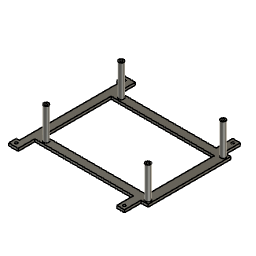
PCB_Rev1_Holder v4 (Autodesk Fusion 360 design; units mm, degrees)
Autodesk Fusion 360 part; units mm, degrees
note: some values were not read from the file. Set by a fixed rule: which face or edge a step refers to.
sketch "Sketch1" plane through (0, 0, 0) normal (0, 0, 1) x (1, 0, 0)
  line L0 (0, 180) -> (180, 180)
  line L1 (180, 180) -> (180, 0)
  line L2 (180, 0) -> (0, 0)
  line L3 (0, 0) -> (0, 180)
  line L4 (10, 170) -> (170, 170)
  line L5 (170, 170) -> (170, 10)
  line L6 (170, 10) -> (10, 10)
  line L7 (10, 10) -> (10, 170)
  constraint horizontal L0
  constraint vertical L1
  constraint horizontal L2
  constraint vertical L3
  constraint horizontal L4
  constraint vertical L5
  constraint horizontal L6
  constraint vertical L7
sketch "Sketch2" plane through (0, 0, 4) normal (0, 0, 1) x (-1, 0, 0)
  line L0 (-170, -10) -> (-10, -10)
  line L1 (-10, -10) -> (-10, -170)
  line L2 (-10, -170) -> (-170, -170)
  line L3 (-170, -170) -> (-170, -10)
  line L4 (0, 0) -> (-180, 0)
  line L5 (-180, 0) -> (-180, -180)
  line L6 (-180, -180) -> (0, -180)
  line L7 (0, -180) -> (0, 0)
  circle A0 centre (-5, -5) radius 2
sketch "Sketch3" plane through (0, 0, 0) normal (0, 0, 1) x (1, 0, 0)
  line L0 (0, 0) -> (172, 0)
  line L1 (172, 0) -> (172, 130)
  line L2 (172, 130) -> (0, 130)
  line L3 (0, 130) -> (0, 0)
  line L4 (12, 12) -> (158, 12)
  line L5 (158, 12) -> (158, 118)
  line L6 (158, 118) -> (12, 118)
  line L7 (12, 118) -> (12, 12)
  dimension "d5" = 172
  dimension "d6" = 130
  constraint horizontal L0
  constraint vertical L1
  constraint horizontal L2
  constraint vertical L3
  constraint coincident L0.start L3.end
  constraint horizontal L4
  constraint vertical L5
  constraint horizontal L6
  constraint vertical L7
  measures "d5" distance of L0.start L0.end
  measures "d6" distance of L0.start L2.end
extrude "Extrude3" add sketch "Sketch3" along normal blind 4
sketch "Sketch4" plane through (0, 0, 4) normal (0, 0, 1) x (-1, 0, 0)
  line L0 (-12, -12) -> (-12, -118)
  line L1 (-12, -118) -> (-158, -118)
  line L2 (-158, -118) -> (-158, -12)
  line L3 (-158, -12) -> (-12, -12)
  line L4 (0, -130) -> (0, 0)
  line L5 (0, 0) -> (-172, 0)
  line L6 (-172, 0) -> (-172, -130)
  line L7 (-172, -130) -> (0, -130)
  circle A0 centre (-6, -6) radius 4
extrude "Extrude4" add sketch "Sketch4" along normal blind 10 contours A0
sketch "Sketch5" plane through (0, 0, 4) normal (0, 0, 1) x (-1, 0, 0)
  circle A0 centre (-6, -6) radius 4
  line L0 (-12, -12) -> (-12, -118)
  line L1 (-12, -118) -> (-158, -118)
  line L2 (-158, -118) -> (-158, -12)
  line L3 (-158, -12) -> (-12, -12)
  line L4 (0, -130) -> (0, 0)
  line L5 (0, 0) -> (-172, 0)
  line L6 (-172, 0) -> (-172, -130)
  line L7 (-172, -130) -> (0, -130)
  circle A1 centre (-6, -124) radius 4
extrude "Extrude5" add sketch "Sketch5" along normal blind 10 contours A1
sketch "Sketch6" plane through (0, 0, 0) normal (0, 0, 1) x (1, 0, 0)
sketch "Sketch7" plane through (0, 0, 4) normal (0, 0, 1) x (-1, 0, 0)
  circle A0 centre (-6, -124) radius 4
  circle A1 centre (-6, -6) radius 4
  line L0 (-12, -12) -> (-12, -118)
  line L1 (-12, -118) -> (-158, -118)
  line L2 (-158, -118) -> (-158, -12)
  line L3 (-158, -12) -> (-12, -12)
  line L4 (0, -130) -> (0, 0)
  line L5 (0, 0) -> (-172, 0)
  line L6 (-172, 0) -> (-172, -130)
  line L7 (-172, -130) -> (0, -130)
  circle A2 centre (-166, -124) radius 4
extrude "Extrude6" add sketch "Sketch7" along normal blind 10 contours A2
sketch "Sketch8" plane through (0, 0, 4) normal (0, 0, 1) x (-1, 0, 0)
  circle A0 centre (-166, -124) radius 4
  circle A1 centre (-6, -124) radius 4
  circle A2 centre (-6, -6) radius 4
  line L0 (-12, -12) -> (-12, -118)
  line L1 (-12, -118) -> (-158, -118)
  line L2 (-158, -118) -> (-158, -12)
  line L3 (-158, -12) -> (-12, -12)
  line L4 (0, -130) -> (0, 0)
  line L5 (0, 0) -> (-172, 0)
  line L6 (-172, 0) -> (-172, -130)
  line L7 (-172, -130) -> (0, -130)
  circle A3 centre (-166, -6) radius 4
extrude "Extrude7" add sketch "Sketch8" along normal blind 10 contours A3
sketch "Sketch9" plane through (0, 0, 0) normal (0, 0, 1) x (1, 0, 0)
  line L0 (0, 0) -> (10, 0)
  line L1 (10, 0) -> (10, -26)
  line L2 (10, -26) -> (0, -26)
  line L3 (0, -26) -> (0, 0)
  constraint horizontal L0
  constraint vertical L1
  constraint horizontal L2
  constraint vertical L3
  constraint coincident L0.start L3.end
extrude "Extrude8" add sketch "Sketch9" along normal blind 4
sketch "Sketch10" plane through (0, 0, 0) normal (0, 0, 1) x (1, 0, 0)
  line L0 (172, 0) -> (160, 0)
  line L1 (160, 0) -> (160, -26)
  line L2 (160, -26) -> (172, -26)
  line L3 (172, -26) -> (172, 0)
  constraint horizontal L0
  constraint vertical L1
  constraint horizontal L2
  constraint vertical L3
extrude "Extrude9" add sketch "Sketch10" along normal blind 4
sketch "Sketch11" plane through (0, 0, 0) normal (0, 0, 1) x (1, 0, 0)
  line L0 (0, 130) -> (12, 130)
  line L1 (12, 130) -> (12, 156)
  line L2 (12, 156) -> (0, 156)
  line L3 (0, 156) -> (0, 130)
  line L4 (172, 130) -> (160, 130)
  line L5 (160, 130) -> (160, 156)
  line L6 (160, 156) -> (172, 156)
  line L7 (172, 156) -> (172, 130)
  constraint horizontal L0
  constraint vertical L1
  constraint horizontal L2
  constraint vertical L3
  constraint horizontal L4
  constraint vertical L5
  constraint horizontal L6
  constraint vertical L7
extrude "Extrude10" add sketch "Sketch11" along normal blind 4
sketch "Sketch12" plane through (0, 0, 0) normal (0, 0, 1) x (1, 0, 0)
  line L0 (0, -26, 4) -> (-5, -26, 4)
  line L1 (-5, -26, 4) -> (-5, -14, 4)
  line L2 (-5, -14, 4) -> (0, -14, 4)
  line L3 (0, -14, 4) -> (0, -26, 4)
  line L4 (172, -26, 4) -> (177, -26, 4)
  line L5 (177, -26, 4) -> (177, -14, 4)
  line L6 (177, -14, 4) -> (172, -14, 4)
  line L7 (172, -14, 4) -> (172, -26, 4)
  line L8 (172, 156, 4) -> (177, 156, 4)
  line L9 (177, 156, 4) -> (177, 144, 4)
  line L10 (177, 144, 4) -> (172, 144, 4)
  line L11 (172, 144, 4) -> (172, 156, 4)
  line L12 (0, 156, 4) -> (-5, 156, 4)
  line L13 (-5, 156, 4) -> (-5, 144, 4)
  line L14 (-5, 144, 4) -> (0, 144, 4)
  line L15 (0, 144, 4) -> (0, 156, 4)
extrude "Extrude11" add sketch "Sketch12" against normal blind 4 contours L0 L1 L2 L3 | L4 L5 L6 L7 | L8 L9 L10 L11 | L12 L13 L14 L15 in plane through (0, 0, 4) normal (0, 0, 1)
sketch "Sketch13" plane through (0, 0, 0) normal (0, 0, -1) x (1, 0, 0)
  line L0 (12, -118) -> (12, -12)
  line L1 (12, -12) -> (158, -12)
  line L2 (158, -12) -> (158, -118)
  line L3 (158, -118) -> (12, -118)
  line L4 (-5, -156) -> (12, -156)
  line L5 (12, -156) -> (12, -130)
  line L6 (12, -130) -> (160, -130)
  line L7 (160, -130) -> (160, -156)
  line L8 (160, -156) -> (177, -156)
  line L9 (177, -156) -> (177, -144)
  line L10 (177, -144) -> (172, -144)
  line L11 (172, -144) -> (172, -130)
  line L12 (172, -130) -> (172, 0)
  line L13 (172, 0) -> (172, 14)
  line L14 (172, 14) -> (177, 14)
  line L15 (177, 14) -> (177, 26)
  line L16 (177, 26) -> (160, 26)
  line L17 (160, 26) -> (160, 0)
  line L18 (160, 0) -> (10, 0)
  line L19 (10, 0) -> (10, 26)
  line L20 (10, 26) -> (-5, 26)
  line L21 (-5, 26) -> (-5, 14)
  line L22 (-5, 14) -> (0, 14)
  line L23 (0, 14) -> (0, -144)
  line L24 (0, -144) -> (-5, -144)
  line L25 (-5, -144) -> (-5, -156)
  circle A0 centre (1, 20) radius 2
  circle A1 centre (171, 20) radius 2
extrude "Extrude12" cut sketch "Sketch13" against normal blind 4 contours A0 | A1
sketch "Sketch14" plane through (0, 0, 4) normal (0, 0, 1) x (-1, 0, 0)
  circle A0 centre (-1, 20) radius 2
  circle A1 centre (-171, 20) radius 2
  circle A2 centre (-166, -6) radius 4
  circle A3 centre (-166, -124) radius 4
  circle A4 centre (-6, -124) radius 4
  circle A5 centre (-6, -6) radius 4
  line L0 (-12, -12) -> (-12, -118)
  line L1 (-12, -118) -> (-158, -118)
  line L2 (-158, -118) -> (-158, -12)
  line L3 (-158, -12) -> (-12, -12)
  line L4 (0, -144) -> (0, 14)
  line L5 (0, 14) -> (5, 14)
  line L6 (5, 14) -> (5, 26)
  line L7 (5, 26) -> (-10, 26)
  line L8 (-10, 26) -> (-10, 0)
  line L9 (-10, 0) -> (-160, 0)
  line L10 (-160, 0) -> (-160, 26)
  line L11 (-160, 26) -> (-177, 26)
  line L12 (-177, 26) -> (-177, 14)
  line L13 (-177, 14) -> (-172, 14)
  line L14 (-172, 14) -> (-172, 0)
  line L15 (-172, 0) -> (-172, -130)
  line L16 (-172, -130) -> (-172, -144)
  line L17 (-172, -144) -> (-177, -144)
  line L18 (-177, -144) -> (-177, -156)
  line L19 (-177, -156) -> (-160, -156)
  line L20 (-160, -156) -> (-160, -130)
  line L21 (-160, -130) -> (-12, -130)
  line L22 (-12, -130) -> (-12, -156)
  line L23 (-12, -156) -> (5, -156)
  line L24 (5, -156) -> (5, -144)
  line L25 (5, -144) -> (0, -144)
  circle A6 centre (-1, -150) radius 2
  circle A7 centre (-171, -150) radius 2
extrude "Extrude13" cut sketch "Sketch14" against normal blind 4 contours A6 | A7
extrude "Extrude14" add 4 faces at (166.0996, 8.1156, 14) (167.2013, 123.4215, 14) (6.6074, 6.7617, 14) (7.1017, 125.1485, 14) along direction (0, 0, 1) blind 40
sketch "Sketch15" plane through (0, 0, 54) normal (0, 0, 1) x (-1, 0, 0)
  circle A0 centre (-166, -6) radius 4
  circle A1 centre (-166, -6) radius 2
  circle A2 centre (-166, -124) radius 2
  circle A3 centre (-6, -124) radius 2
  circle A4 centre (-6, -6) radius 2
  constraint concentric A0 A1
extrude "Extrude15" cut sketch "Sketch15" against normal blind 14 contours A1 | A2 | A3 | A4
move_face "OffsetFaces1" offset 16 3 faces at (172, -9.3333, 1.3333) (172, 43.3333, 2.6667) (172, 139.3333, 1.3333)
extrude "Extrude16" cut 1 faces at (158, 47.3333, 2.6667) along direction (1, 0, 0) blind 16
move_face "MoveFace1" to x (1, 0, 0) y (0, 1, 0) z (0, 0, 1) at (16, 0, 0) 2 faces at (165.3054, 120.0608, 20.6667) (164.4679, 122.7144, 44.6667)
move_face "MoveFace2" to x (1, 0, 0) y (0, 1, 0) z (0, 0, 1) at (16, 0, 0) 6 faces at (4.0099, 124.1991, 44.6667) (8.7929, 126.8635, 37.3333) (2.0199, 6.3983, 20.6667) (4.0099, 6.1991, 44.6667) (165.1774, 4.177, 44.6667) (165.5026, 9.969, 37.3333)
extrude "Extrude17" cut 2 faces at (160, 138.6667, 1.3333) (160, -8.6667, 1.3333) along direction (1, 0, 0) blind 4
extrude "Extrude18" cut 2 faces at (164, -8.6667, 1.3333) (164, 138.6667, 1.3333) along direction (1, 0, 0) blind 1
extrude "Extrude19" cut 1 faces at (180.6667, 144, 2.6667) along direction (0, -1, 0) blind 16
extrude "Extrude20" add 1 faces at (182.3333, 128, 1.3333) along direction (0, 1, 0) blind 2
extrude "Extrude21" cut 1 faces at (180.6667, -14, 2.6667) along direction (0, 1, 0) blind 14
